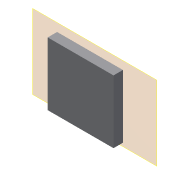
# Autodesk Inventor part: cellSTORM_Flipmirror
Saved by Autodesk Inventor 2022 (Build 260153000, 153)
## iProperties
Created: 2022-06-23
Part Number: cellSTORM_Flipmirror
Material: Generisch
Document SubType Name: Modeling
Designer: Muriel
Density: 1 g/cm^3
Appearance: Vorgabe
Author: Muriel
Autodesk Inventor part; units mm, degrees
ref_plane "YZ Plane" through (0, 0, 0) normal (1, 0, 0) x (0, 1, 0)
ref_plane "XZ Plane" through (0, 0, 0) normal (0, 1, 0) x (-1, 0, 0)
ref_plane "XY Plane" through (0, 0, 0) normal (0, 0, 1) x (1, 0, 0)
ref_plane "Arbeitsebene1" through (0, 0, 4) normal (0, 0, 1) x (1, 0, 0)
sketch "Skizze1" plane through (0, 0, 4) normal (0, 0, 1) x (1, 0, 0)
  circle A0 centre (33.0405, -20.0687) radius 1.4 projected
  circle A1 centre (15.72, -10.0687) radius 1.4 projected
  circle A2 centre (15.72, -30.0687) radius 1.4 projected
  line L0 (0, -18.4687) -> (28.3951, -18.4687) projected
  arc A3 (28.3951, -21.6687) -> (28.3951, -18.4687) centre (28.3951, -20.0687) ccw projected
  line L1 (28.3951, -21.6687) -> (0, -21.6687) projected
  line L2 (0, -36.0687) -> (0, -21.6687) projected
  line L3 (0, -36.0687) -> (55, -36.0687) projected
  line L4 (55, -36.0687) -> (55, -6.0687) projected
  line L5 (55, -6.0687) -> (60, -6.0687) projected
  line L6 (60, 0) -> (60, -6.0687) projected
  line L7 (0, 0) -> (60, 0) projected
  line L8 (0, -18.4687) -> (0, 0) projected
  line L9 (12.5, -35.0687) -> (42.5, -35.0687)
  line L10 (42.5, -35.0687) -> (42.5, -5.0687)
  line L11 (42.5, -5.0687) -> (12.5, -5.0687)
  line L12 (12.5, -5.0687) -> (12.5, -35.0687)
  line L13 (12.5, -35.0687) -> (42.5, -5.0687) construction
  line L14 (42.5, -35.0687) -> (12.5, -5.0687) construction
  circle A4 centre (33.0405, -20.0687) radius 2.45
  circle A5 centre (15.72, -10.0687) radius 2.45
  circle A6 centre (15.72, -30.0687) radius 2.45
  line L15 (12.5, -18.4687) -> (12.5, -21.6687)
  point P0 (27.5, -20.0687)
  point P1 (18.7387, -21.6687)
  point P2 (11.6841, -36.0687)
  point P3 (46.6841, -36.0687)
  point P4 (18.7387, -18.4687)
  dimension "d0" = 30
  dimension "d1" = 30
  dimension "d2" = 4.9
  dimension "d3" = 4.9
  dimension "d4" = 4.9
  constraints: 14 end point, 4 point on line, 3 centre point, 3 coincident, 2 midpoint, 2 parallel, 1 horizontal, 1 perpendicular
  measures "d0" distance of L11.end L10.end
  measures "d1" distance of L10.end L9.end
  measures "d2" diameter of A4
  measures "d3" diameter of A5
  measures "d4" diameter of A6
extrude "Extrusion1" add sketch "Skizze1" along normal blind 4 contours L12 L11 L10 L9 L1 A3 L0 | L0 A3 L1 L12
sketch "Skizze2" plane through (0, 0, 8) normal (0, 0, 1) x (1, 0, 0)
  line L0 (12.5, -5.0687) -> (12.5, -35.0687) projected
  line L1 (42.5, -35.0687) -> (42.5, -5.0687) projected
  line L2 (42.5, -5.0687) -> (12.5, -5.0687) projected
  circle A0 centre (33.0405, -20.0687) radius 2.45 projected
  line L3 (12.5, -35.0687) -> (42.5, -35.0687) projected
  point P0 (0, 0)
extrude "Extrusion2" add sketch "Skizze2" along normal blind 1 contours L2 L1 L3 L0 | A0
sketch "Skizze3" plane through (0, 0, 9) normal (0, 0, 1) x (1, 0, 0)
  line L0 (12.5, -35.0687) -> (42.5, -35.0687) projected
  line L1 (42.5, -35.0687) -> (42.5, -5.0687) projected
  line L2 (42.5, -5.0687) -> (12.5, -5.0687) projected
  line L3 (12.5, -5.0687) -> (12.5, -35.0687) projected
  line L4 (37.9557, 14.9579) -> (17.8567, -20.2718) projected
  line L5 (17.8567, -20.2718) -> (-3.0822, -20.2721) projected
  line L6 (15.4322, -16.0975) -> (22.0334, -27.4633)
  line L7 (12.5, -5.0687) -> (12.5, -35.0687) projected
  line L8 (12.5, -23.3829) -> (44.0331, -5.0687)
  line L9 (42.5, -35.0687) -> (42.5, -5.0687) projected
  line L10 (42.5, -5.9591) -> (42.5, -10.9591)
  line L11 (42.5, -10.9591) -> (12.5, -28.3829)
  point P0 (0, 0)
  point P1 (42.5, -5.9591)
  point P2 (12.5, -28.3829)
  dimension "d9" = 119.706
  dimension "d10" = 59.853
  dimension "d11" = 5
  constraints: 8 end point, 8 point on line, 1 parallel, 1 perpendicular
  measures "d9" angle of L5 L4
  measures "d10" angle of L6 L4
  measures "d11" distance of L10.start L10.end
extrude "Extrusion3" add sketch "Skizze3" along normal blind 20 contours L3 L8 L6 L11 | L11 L6 L8 L1
equation "\"d10\" = 0.5 * d9"
